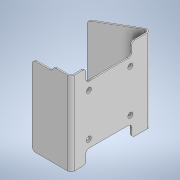
# Autodesk Inventor part: armor
Saved by Autodesk Inventor 2021 (Build 250183000, 183)
## iProperties
Created: 2022-05-14
Part Number: armor
Material: Generic
Document SubType Name: Modeling
Designer: ermoz
Density: 1 g/cm^3
Appearance: Default
Author: ermoz
Autodesk Inventor part; units mm, degrees
ref_plane "YZ Plane" through (0, 0, 0) normal (1, 0, 0) x (0, 1, 0)
ref_plane "XZ Plane" through (0, 0, 0) normal (0, 1, 0) x (-1, 0, 0)
ref_plane "XY Plane" through (0, 0, 0) normal (0, 0, 1) x (1, 0, 0)
sketch "Sketch2" plane through (0, 0, 0) normal (0, 1, 0) x (-1, 0, 0)
  line L0 (-23.5, 25.6213) -> (-23.5, 95)
  line L1 (-23.5, 95) -> (-25, 95)
  line L2 (-25, 95) -> (-25, 25)
  line L3 (-25, 25) -> (0, 0)
  line L4 (0, 0) -> (25, 25)
  line L5 (23.5, 25.6213) -> (0, 2.1213)
  line L6 (0, 2.1213) -> (-23.5, 25.6213)
  line L7 (23.5, 25.6213) -> (25, 25)
  line L8 (25, 25) -> (-25, -3.8675)
  line L9 (-25, -3.8675) -> (-25, 25)
  line L10 (-23.5, 25.6213) -> (-23.5, -1.2694)
  line L11 (-23.5, -1.2694) -> (24.25, 26.299)
  line L12 (24.25, 26.299) -> (25, 25)
  point P0 (24.5092, 24.5092)
  dimension "d11" = 1.5
  dimension "d18" = 1.5
  dimension "d19" = 1.5
  dimension "d27" = 70
  dimension "d28" = 50
  dimension "d29" = 135
  dimension "d47" = 60
  dimension "d48" = 1.5
  constraints: 26 end point, 7 perpendicular, 3 vertical, 2 parallel, 1 coincident
  measures "d11" distance of L0.end L1.end
  measures "d18" distance between parallel lines of L6 L3
  measures "d19" distance between parallel lines of L4 L5
  measures "d27" distance of L1.end L2.end
  measures "d28" distance of L2.end L4.end
  measures "d29" angle of L0 L6
  measures "d47" angle of L8 L9
  measures "d48" distance between parallel lines of L8 L11
extrude "Extrusion2" add sketch "Sketch2" along normal blind 100 contours L10 L3 L2 L1 L0 | L11 L12 L7 L5 L8 L6 | L6 L8 L3 L11 | L10 L11 L3 L8 L9 | L5 L7 L8
fillet "Fillet3" radius 2.5 1 edges at (23.5, 50, -1.2694)
sketch "Sketch7" plane through (23.5, 0, 95) normal (-1, 0, 0) x (0, 0, 1)
  line L0 (0, 0) -> (0, 100) projected
  line L1 (0, 0) -> (-1.5, 0)
  line L2 (-1.5, 0) -> (-1.5, 100)
  line L3 (-1.5, 100) -> (0, 100)
  line L4 (0, 100) -> (0, 0)
  line L5 (-91.9393, 100) -> (0, 100) projected
  point P0 (-95, 0)
  dimension "d49" = 1.5
  constraints: 8 end point, 2 parallel, 1 collinear, 1 horizontal, 1 perpendicular
  measures "d49" distance between parallel lines of L0 L2
extrude "Extrusion7" add sketch "Sketch7" along normal blind 45
fillet "Fillet12" radius 4 2 edges at (25, 50, 95) (25, 50, -3.8675)
fillet "Fillet13" radius 2.5 1 edges at (23.5, 50, 93.5)
sketch "Sketch8" plane through (23.5, 0, 3.0607) normal (-1, 0, 0) x (0, 0, 1)
  line L0 (18.9393, 0) -> (73.9393, 0)
  line L1 (73.9393, 0) -> (73.9393, 15)
  line L2 (73.9393, 15) -> (18.9393, 15)
  line L3 (18.9393, 15) -> (18.9393, 0)
  line L4 (18.9393, 85) -> (73.9393, 85)
  line L5 (73.9393, 85) -> (73.9393, 100)
  line L6 (73.9393, 100) -> (18.9393, 100)
  line L7 (18.9393, 100) -> (18.9393, 85)
  line L8 (0, 100) -> (87.9393, 100) projected
  line L9 (0, 0) -> (87.9393, 0) projected
  line L10 (91.9393, 0) -> (91.9393, 100) projected
  point P0 (-3.0607, 0)
  dimension "d54" = 15
  dimension "d55" = 55
  dimension "d58" = 18
  constraints: 16 end point, 4 parallel, 3 collinear, 2 horizontal, 2 perpendicular, 2 point on line
  measures "d54" distance of L0.end L1.end
  measures "d55" distance of L0.start L0.end
  measures "d58" distance between parallel lines of L10 L1
extrude "Extrusion8" cut sketch "Sketch8" against normal through all
sketch "Sketch9" plane through (-21.5, 0, 95) normal (0, 0, 1) x (1, 0, 0)
  line L0 (0, 100) -> (0, 0) projected
  line L1 (0, 100) -> (25, 100)
  line L2 (25, 100) -> (25, 95)
  line L3 (25, 95) -> (0, 95)
  line L4 (0, 95) -> (0, 100)
  point P0 (21.5, 0)
  dimension "d60" = 5
  dimension "d61" = 25
  constraints: 8 end point, 2 parallel, 1 horizontal, 1 perpendicular
  measures "d60" distance of L1.end L2.end
  measures "d61" distance of L0.start L1.end
extrude "Extrusion9" cut sketch "Sketch9" against normal blind 35
fillet "Fillet14" radius 4 14 edges at (24.25, 85, 77) (24.25, 85, 22) (24.25, 100, 22) (24.25, 100, 77) (24.25, 15, 22) (24.25, 0, 22) (24.25, 15, 77) (24.25, 0, 77) (-21.5, 95, 94.25) (3.5, 95, 94.25) (3.5, 100, 94.25) (-21.5, 0, 94.25) (-24.625, 0, 25.6495) (-24.625, 100, 25.6495)
sketch "Sketch10" plane through (25, 0, 3.0607) normal (1, 0, 0) x (0, 0, -1)
  circle A0 centre (-70.4393, 75.5) radius 1.5
  circle A1 centre (-20.4393, 75.5) radius 1.5
  circle A2 centre (-70.4393, 24.5) radius 1.5
  circle A3 centre (-20.4393, 24.5) radius 1.5
  line L0 (-91.9393, 100) -> (-91.9393, 0) projected
  line L1 (-91.9393, 4) -> (-91.9393, 91) projected
  line L2 (-87.9393, 100) -> (-77.9393, 100) projected
  point P0 (3.0607, 0)
  dimension "d64" = 3
  dimension "d65" = 50
  dimension "d66" = 51
  dimension "d70" = 24.5
  dimension "d71" = 21.5
  constraints: 4 centre point, 3 equal radius, 2 horizontal alignment, 2 vertical alignment
  measures "d64" diameter of A1
  measures "d65" distance of A1.centre A0.centre
  measures "d66" distance of A0.centre A2.centre
  measures "d70" distance from line of L2 A0.centre
  measures "d71" distance from line of L0 A0.centre
extrude "Extrusion10" cut sketch "Sketch10" against normal blind 5
chamfer "Chamfer1" distance 1.5 angle 45 4 edges at (25, 75.5, 75) (25, 75.5, 25) (25, 24.5, 25) (25, 24.5, 75)
body "Solid2"
